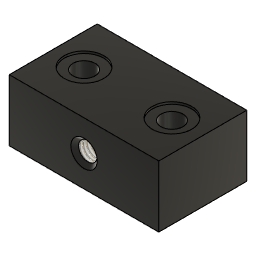
Door Opener Mechanism (Autodesk Fusion 360 archive; units mm, degrees)
design "BoxBracket"
Autodesk Fusion 360 part; units mm, degrees
sketch "Sketch1" plane through (0, 0, 0) normal (0, 0, 1) x (1, 0, 0) in component "BoxBracket"
  line L0 (0, 0) -> (34, 0)
  line L1 (34, 0) -> (34, 20)
  line L2 (34, 20) -> (0, 20)
  line L3 (0, 20) -> (0, 0)
  circle A0 centre (27, 10) radius 2.5
  circle A1 centre (7, 10) radius 2.5
  line L4 (0, 10) -> (34, 10) construction
  circle A2 centre (7, 10) radius 4.5
  circle A3 centre (27, 10) radius 4.5
  line L5 (11, 12.3094) -> (7, 14.6188)
  line L6 (7, 14.6188) -> (3, 12.3094)
  line L7 (3, 12.3094) -> (3, 7.6906)
  line L8 (3, 7.6906) -> (7, 5.3812)
  line L9 (7, 5.3812) -> (11, 7.6906)
  line L10 (11, 7.6906) -> (11, 12.3094)
  line L11 (23, 7.6906) -> (27, 5.3812)
  line L12 (27, 5.3812) -> (31, 7.6906)
  line L13 (31, 7.6906) -> (31, 12.3094)
  line L14 (31, 12.3094) -> (27, 14.6188)
  line L15 (27, 14.6188) -> (23, 12.3094)
  line L16 (23, 12.3094) -> (23, 7.6906)
  point P0 (17, 10)
  point P1 (7, 10)
  point P2 (27, 10)
  dimension "d1" = 34
  dimension "d2" = 20
  dimension "d3" = 5
  dimension "d4" = 5
  dimension "d5" = 20
  dimension "d6" = 10
  dimension "d7" = 9
  dimension "d8" = 9
  dimension "d9" = 4
  dimension "d10" = 4
  constraint horizontal L0
  constraint vertical L1
  constraint horizontal L2
  constraint vertical L3
  constraint coincident L0.start L3.end
  constraint midpoint L3 L4.start
  constraint midpoint L1 L4.end
  constraint coincident P2 L4
  constraint coincident P1 L4
  constraint midpoint L4 P0
  constraint concentric A1 A2
  constraint concentric A0 A3
  constraint coincident P1 A1.centre
  constraint vertical L10
  constraint coincident P2 A0.centre
  constraint vertical L16
  measures "d1" distance of L0.start L0.end
  measures "d2" distance of L0.start L2.end
  measures "d3" diameter of A0
  measures "d4" diameter of A1
  measures "d5" distance of P2 P1
  measures "d6" distance of P2 P0
  measures "d7" diameter of A2
  measures "d8" diameter of A3
  measures "d9" distance of P1 L10
  measures "d10" distance of P2 L16
extrude "Extrude1" add sketch "Sketch1" along normal blind 14 contours L0 L1 L2 L3 | A2 L10 | A2 L5 L6 L7 L8 L9 L10 | A2 L5 L10 | A2 L9 L10 | A2 L5 | A2 L9 | A2 L5 L6 | A2 L8 L9 | A2 L6 | A2 L8 | A2 L6 L7 | A2 L7 L8 | A2 L7 | A3 L13 | A3 L11 L12 L13 L14 L15 L16 | A3 L13 L14 | A3 L12 L13 | A3 L14 | A3 L12 | A3 L14 L15 | A3 L11 L12 | A3 L15 | A3 L11 | A3 L15 L16 | A3 L11 L16 | A3 L16 in component "BoxBracket"
extrude "Extrude2" cut sketch "Sketch1" along normal blind 5 contours A2 L5 L6 L7 L8 L9 L10 | A2 L5 L10 | A2 L9 L10 | A2 L5 L6 | A2 L8 L9 | A2 L6 L7 | A2 L7 L8 | A3 L11 L12 L13 L14 L15 L16 | A3 L13 L14 | A3 L12 L13 | A3 L14 L15 | A3 L11 L12 | A3 L15 L16 | A3 L11 L16 in component "BoxBracket"
extrude "Extrude3" cut sketch "Sketch1" against normal blind 0.5 from surface at 14 contours A2 L10 | A2 L5 L6 L7 L8 L9 L10 | A2 L5 | A2 L9 | A2 L6 | A2 L8 | A2 L7 | A3 L13 | A3 L11 L12 L13 L14 L15 L16 | A3 L14 | A3 L12 | A3 L15 | A3 L11 | A3 L16 in component "BoxBracket"
sketch "Sketch2" plane through (0, 0, 0) normal (0, -1, 0) x (1, 0, 0) in component "BoxBracket"
  line L0 (0, 0) -> (34, 0)
  line L1 (34, 0) -> (34, 14)
  line L2 (34, 14) -> (0, 14)
  line L3 (0, 14) -> (0, 0)
  line L4 (17, 14) -> (17, 0) construction
  circle A0 centre (17, 7) radius 2.5
  dimension "d18" = 5
  constraint midpoint L2 L4.start
  constraint midpoint L0 L4.end
  constraint midpoint L4 A0.centre
  measures "d18" diameter of A0
hole "Hole1" at (17, 0, 7) direction (0, 1, 0) diameter 4.234 depth 21 tip angle 118 countersink diameter 6 countersink angle 90 in component "BoxBracket"
thread "Thread1" "ISO Metric profile 5.0 M5x0.8 6H" major diameter 5.12 minor diameter 4.234 pitch 0.8 angle 60 resizes the face on face at (17.2108, 13.6277, 4.8935) in component "BoxBracket"
chamfer "Chamfer1" distance 1 angle 45 1 edges at (16.2345, 20, 8.9737) in component "BoxBracket"
component "BoxBracket" placed x (1, 0, 0) y (0, 1, 0) z (0, 0, 1) at (0, 0, 0)
equation "d1 = BoxBracketLength"
equation "d2 = BoxBracketWidth"
equation "d11 = BoxBracketHeight"
equation "BoxBracketWidth = 20 mm"
equation "BoxBracketLength = 34 mm"
equation "BoxBracketHeight = 14 mm"
named bodies: "Box Bracket"

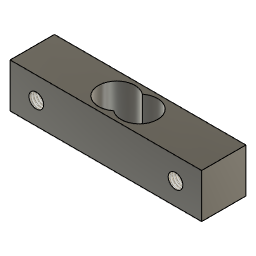
design "Strain Gauge 5Kg"
Autodesk Fusion 360 part; units mm, degrees
sketch "Sketch1" plane through (0, 0, 0) normal (0, 0, 1) x (1, 0, 0) in component "Strain Gauge"
  line L0 (0, 0) -> (55, 0)
  line L1 (55, 0) -> (55, 12.7)
  line L2 (55, 12.7) -> (0, 12.7)
  line L3 (0, 12.7) -> (0, 0)
  circle A0 centre (24.25, 6.35) radius 5.25
  line L4 (0, 6.35) -> (24.25, 6.35) construction
  line L5 (27.5, 12.7) -> (27.5, 0) construction
  circle A1 centre (30.75, 6.35) radius 5.25
  dimension "d1" = 55
  dimension "d2" = 12.7
  dimension "d3" = 10.5
  dimension "d4" = 24.25
  constraint horizontal L0
  constraint vertical L1
  constraint horizontal L2
  constraint vertical L3
  constraint coincident L0.start L3.end
  constraint midpoint L3 L4.start
  constraint perpendicular L3 L4
  constraint coincident A0.centre L4.end
  constraint midpoint L2 L5.start
  constraint midpoint L0 L5.end
  constraint symmetric A0 L5 A1
  measures "d1" distance of L0.start L0.end
  measures "d2" distance of L0.start L2.end
  measures "d3" diameter of A0
  measures "d4" distance of L4.start A0.centre
extrude "Extrude1" add sketch "Sketch1" along normal blind 12.7 in component "Strain Gauge"
sketch "Sketch2" plane through (0, 0, 0) normal (0, -1, 0) x (1, 0, 0) in component "Strain Gauge"
  line L0 (0, 0) -> (55, 0)
  line L1 (55, 0) -> (55, 12.7)
  line L2 (55, 12.7) -> (0, 12.7)
  line L3 (0, 12.7) -> (0, 0)
  line L4 (7.5, 6.35) -> (47.5, 6.35) construction
  line L5 (27.5, 6.35) -> (27.5, 12.7) construction
  line L6 (47.5, 6.35) -> (55, 6.35) construction
  dimension "d7" = 40
  constraint horizontal L4
  constraint midpoint L4 L5.start
  constraint midpoint L2 L5.end
  constraint vertical L5
  constraint midpoint L1 L6.end
  constraint horizontal L6
  measures "d7" distance of L4.start L4.end
hole "Hole1" at (7.5, 0, 6.35) direction (0, 1, 0) diameter 4.234 depth 15 tip angle 118 in component "Strain Gauge"
thread "Thread1" "ISO Metric profile 5.0 M5x0.8 6H" thread offset 0 thread depth 7.4 in component "Strain Gauge"
hole "Hole2" at (47.5, 0, 6.35) direction (0, 1, 0) diameter 4.234 depth 26 tip angle 118 in component "Strain Gauge"
thread "Thread2" "ISO Metric profile 5.0 M5x0.8 6H" thread offset 0 thread depth 7.4 in component "Strain Gauge"
component "Strain Gauge" placed x (1, 0, 0) y (0, 1, 0) z (0, 0, 1) at (0, 0, 0)
equation "d4 = 19 mm + ( 10.5 / 2 ) * 1 mm"

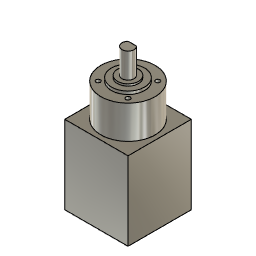
design "StepperMotor17HS19"
Autodesk Fusion 360 part; units mm, degrees
sketch "Sketch1" plane through (0, 0, 0) normal (0, 0, 1) x (1, 0, 0) in component "GearedStepper17HS19"
  line L0 (21, -21) -> (-21, -21)
  line L1 (-21, -21) -> (-21, 21)
  line L2 (-21, 21) -> (21, 21)
  line L3 (21, 21) -> (21, -21)
  line L4 (21, -21) -> (-21, 21) construction
  line L5 (-21, -21) -> (21, 21) construction
  circle A0 centre (0, 0) radius 18
  circle A1 centre (0, 0) radius 11
  circle A2 centre (0, 0) radius 14 construction
  circle A3 centre (9.8995, 9.8995) radius 1.45
  circle A4 centre (-9.8995, 9.8995) radius 1.45
  circle A5 centre (-9.8995, -9.8995) radius 1.45
  circle A6 centre (9.8995, -9.8995) radius 1.45
  circle A7 centre (0, 0) radius 4
  line L6 (-2.755, 2.9) -> (2.755, 2.9)
  line L7 (0, 2.9) -> (0, 0) construction
  circle A8 centre (0, 0) radius 7
  dimension "d1" = 42
  dimension "d2" = 42
  dimension "d3" = 36
  dimension "d4" = 22
  dimension "d8" = 28
  dimension "d9" = 2.9
  dimension "d10" = 2.9
  dimension "d11" = 2.9
  dimension "d12" = 2.9
  dimension "d20" = 8
  dimension "d21" = 2.9
  dimension "d28" = 14
  constraint horizontal L0
  constraint perpendicular L0 L1
  constraint parallel L0 L2
  constraint parallel L1 L3
  constraint coincident L4 A0.centre
  constraint coincident L5 A0.centre
  constraint coincident A0.centre A1.centre
  constraint concentric A0 A1
  constraint coincident L5 A3.centre
  constraint coincident A2 A3.centre
  constraint coincident L4 A4.centre
  constraint coincident A2 A4.centre
  constraint coincident L5 A5.centre
  constraint coincident A2 A5.centre
  constraint coincident L4 A6.centre
  constraint coincident A2 A6.centre
  constraint concentric A1 A7
  constraint coincident A7 L6.start
  constraint coincident A7 L6.end
  constraint horizontal L6
  constraint midpoint L6 L7.start
  constraint concentric A0 A8
  measures "d1" distance of L1.end L2.end
  measures "d2" distance of L0.end L1.end
  measures "d3" diameter of A0
  measures "d4" diameter of A1
  measures "d8" diameter of A2
  measures "d9" diameter of A3
  measures "d10" diameter of A4
  measures "d11" diameter of A5
  measures "d12" diameter of A6
  measures "d20" diameter of A7
  measures "d21" distance of L7.start A0.centre
  measures "d28" diameter of A8
extrude "Extrude1" add sketch "Sketch1" against normal blind 52 contours L0 L1 L2 L3 | A0 | A1 | A3 | A4 | A5 | A6 | A7 L6 | A7 L6 | A8 in component "GearedStepper17HS19"
extrude "Extrude2" add sketch "Sketch1" along normal blind 22 contours A0 | A1 | A7 L6 | A7 L6 | A8 in component "GearedStepper17HS19"
extrude "Extrude3" add sketch "Sketch1" along normal blind 2 from surface at 22 contours A1 | A7 L6 | A7 L6 | A8 in component "GearedStepper17HS19"
extrude "Extrude5" add sketch "Sketch1" along normal blind 1.3 from surface at 24 contours A7 L6 | A7 L6 | A8 in component "GearedStepper17HS19"
extrude "Extrude4" add sketch "Sketch1" along normal blind 20 from surface at 22 contours A7 L6 picked at (0.8284, -0.9868) in component "GearedStepper17HS19"
chamfer "Chamfer1" [rolled back] distance 3 in component "GearedStepper17HS19"
fillet "Fillet1" [rolled back] radius 2 in component "GearedStepper17HS19"
component "GearedStepper17HS19" placed x (1, 0, 0) y (0, 1, 0) z (0, 0, 1) at (0, 0, 0)
equation "d21 = 6.9 mm - 4 mm"
named bodies: "GearedStepper17HS19"

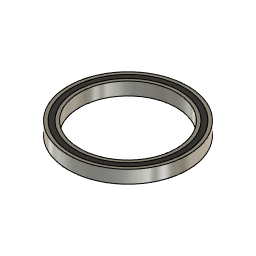
design "Shaft Bearing"
Autodesk Fusion 360 part; units mm, degrees
sketch "Sketch1" plane through (0, 0, 0) normal (0, 0, 1) x (1, 0, 0) in component "Shaft Bearing"
  circle A0 centre (0, 0) radius 15
  circle A1 centre (0, 0) radius 18.5
  circle A2 centre (0, 0) radius 17.5
  circle A3 centre (0, 0) radius 16
  dimension "d4" = 30
  dimension "d5" = 37
  dimension "d6" = -1
  dimension "d7" = 1
  constraint coincident A0.centre A1.centre
  measures "d4" diameter of A0
  measures "d5" diameter of A1
extrude "Extrude1" add sketch "Sketch1" along normal blind 4 contours A1 makes body 1 in component "Shaft Bearing"
extrude "Extrude2" add sketch "Sketch1" along normal blind 4 separate body contours A2 makes body 2 in component "Shaft Bearing"
extrude "Extrude3" add sketch "Sketch1" along normal blind 4 separate body contours A3 makes body 3 in component "Shaft Bearing"
component "Shaft Bearing" placed x (1, 0, 0) y (0, 1, 0) z (0, 0, 1) at (0, 0, 0)
equation "InnerDiam = 30 mm"
equation "OuterDiam = 37 mm"
equation "Thickness = 4 mm"
equation "d4 = InnerDiam"
equation "d5 = OuterDiam"
equation "d8 = Thickness"
equation "d10 = Thickness"
equation "d12 = Thickness"

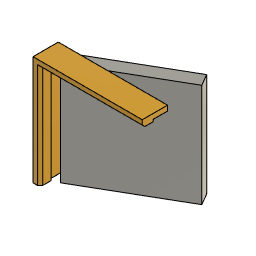
design "Door and Frame"
Autodesk Fusion 360 part; units mm, degrees
sketch "Sketch1" plane through (0, 0, 0) normal (0, 1, 0) x (1, 0, 0) in component "Door Frame"
  line L0 (0, 0) -> (0, 400)
  line L1 (0, 0) -> (400, 0)
  line L2 (-28, -28) -> (-28, 400)
  line L3 (-28, -28) -> (400, -28)
  line L4 (400, 0) -> (400, -28)
  line L5 (0, 400) -> (-28, 400)
  line L6 (-8, -8) -> (400, -8)
  line L7 (-8, -8) -> (-8, 400)
  dimension "d1" = 400
  dimension "d2" = 400
  dimension "d4" = 28
  dimension "d6" = 28
  dimension "d15" = 8
  dimension "d16" = 8
  constraint coincident L0.start L1.start
  constraint vertical L0
  constraint perpendicular L0 L1
  constraint vertical L2
  constraint perpendicular L2 L3
  constraint horizontal L5
  constraint vertical L4
  constraint coincident L4 L6.end
  constraint perpendicular L4 L6
  constraint coincident L5 L7.end
  constraint perpendicular L5 L7
  measures "d1" distance of L0.start L0.end
  measures "d2" distance of L0.start L1.end
  measures "d4" distance of L0 L2
  measures "d6" distance of L1 L3
  measures "d15" distance of L1 L6
  measures "d16" distance of L0 L7
extrude "Extrude1" add sketch "Sketch1" along normal blind 43 makes body 1 in component "Door Frame"
extrude "Extrude1'" add sketch "Sketch1" along normal blind 56 from surface at 43 contours L2 L3 L4 L5 L6 L7 bodies 1 in component "Door Frame"
chamfer "Chamfer1" distance 10 angle 45 2 edges at (0, 0, -200) (200, 0, 0) on bodies 1 in component "Door Frame"
sketch "Sketch1 (2)" plane through (0, 0, 0) normal (0, 1, 0) x (1, 0, 0) in component "Door"
  line L0 (-5, -5) -> (400, -5)
  line L1 (400, -5) -> (400, 400)
  line L2 (400, 400) -> (-5, 400)
  line L3 (-5, 400) -> (-5, -5)
  line L4 (0, 0) -> (400, 0)
  line L5 (0, 0) -> (0, 400)
  line L6 (400, 0) -> (400, -28)
  line L7 (0, 400) -> (-28, 400)
  dimension "d10" = 5
  dimension "d11" = 5
  constraint horizontal L0
  constraint vertical L1
  constraint horizontal L2
  constraint vertical L3
  constraint collinear L1 L6
  constraint collinear L2 L7
  measures "d10" distance of L0 L4
  measures "d11" distance of L3 L5
extrude "Extrude1''" add sketch "Sketch1 (2)" along normal blind 53 from surface at 45 separate body makes body 2 in component "Door"
sketch "Sketch1 (3)" plane through (0, 0, 0) normal (0, 0, 1) x (1, 0, 0) in component "Hinge"
  line L0 (400, 45) -> (-5, 45)
  line L1 (-5, 45) -> (-5, 98)
  line L2 (-28, 0) -> (-28, 99)
  line L3 (-8, 43) -> (-8, 99)
  line L4 (-8, 43) -> (400, 43)
  line L5 (-8, 99) -> (-8, 107)
  line L6 (-8, 107) -> (-5, 107)
  line L7 (-5, 107) -> (-5, 98)
  circle A0 centre (-6.5, 107) radius 7
  line L8 (-8, 107) -> (-11, 107)
  line L9 (-11, 107) -> (-11, 67)
  line L10 (-11, 67) -> (-8, 67)
  line L11 (-8, 67) -> (-8, 107)
  line L12 (-5, 107) -> (-2, 107)
  line L13 (-2, 107) -> (-2, 67)
  line L14 (-2, 67) -> (-5, 67)
  line L15 (-5, 67) -> (-5, 107)
  dimension "d20" = 8
  dimension "d21" = 14
  dimension "d22" = 3
  dimension "d23" = 40
  dimension "d24" = 3
  dimension "d25" = 40
  constraint coincident L3.end L5.start
  constraint parallel L3 L5
  constraint perpendicular L5 L6
  constraint coincident L1.end L7.end
  constraint vertical L7
  constraint midpoint L6 A0.centre
  constraint horizontal L8
  constraint vertical L9
  constraint horizontal L10
  constraint vertical L11
  constraint horizontal L12
  constraint vertical L13
  constraint horizontal L14
  constraint vertical L15
  measures "d20" distance of L3.end L5.end
  measures "d21" diameter of A0
  measures "d22" distance of L5.end L8.end
  measures "d23" distance of L5.end L10.end
  measures "d24" distance of L6.end L12.end
  measures "d25" distance of L6.end L14.end
extrude "Extrude2" add sketch "Sketch1 (3)" against normal blind 80 from surface at -120 contours L6 A0 L8 L9 L12 L13 | L5 A0 L8 L9 L11 | L3 L5 A0 L9 L10 L11 bodies 1 in component "Door Frame"
extrude "Extrude2'" add sketch "Sketch1 (3)" along normal blind 5 from surface at -120 contours L1 L7 A0 L13 L14 L15 | L7 A0 L12 L13 L15 | L6 A0 L8 L9 L12 L13 bodies 2 in component "Door"
component "Door Frame" placed x (1, 0, 0) y (0, 1, 0) z (0, 0, 1) at (0, 0, 0)
component "Door" placed x (1, 0, 0) y (0, 1, 0) z (0, 0, 1) at (0, 0, 0)
component "Hinge" placed x (1, 0, 0) y (0, 1, 0) z (0, 0, 1) at (0, 0, 0)
named bodies: "Frame", "Door"
